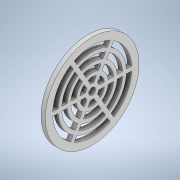
# Autodesk Inventor part: flat drain cover
Saved by Autodesk Inventor 2020.4 (Build 244396000, 396)
## iProperties
Created: 2023-07-18
Part Number: flat drain cover
Material: Generic
Document SubType Name: Modeling
Designer: Paul
Density: 1 g/cm^3
Appearance: Default
Author: Paul
Autodesk Inventor part; units mm, degrees
ref_plane "YZ Plane" through (0, 0, 0) normal (1, 0, 0) x (0, 1, 0)
ref_plane "XZ Plane" through (0, 0, 0) normal (0, 1, 0) x (-1, 0, 0)
ref_plane "XY Plane" through (0, 0, 0) normal (0, 0, 1) x (1, 0, 0)
sketch "Sketch1" plane through (0, 0, 0) normal (0, 1, 0) x (-1, 0, 0)
  line L0 (0, 5.08) -> (0, 10.668)
  line L1 (0, 0) -> (0, 10.668) construction
  line L2 (0, 10.668) -> (0, 18.542)
  line L3 (0, 18.542) -> (0, 24.13)
  line L4 (0, 24.13) -> (0, 32.004)
  line L5 (0, 32.004) -> (0, 37.592)
  line L6 (0, 37.592) -> (0, 45.466)
  line L7 (0, 45.466) -> (0, 51.054)
  line L8 (0, 51.054) -> (0, 58.928)
  line L9 (0, 58.928) -> (0, 66.802)
  line L10 (0, 0) -> (8.7387, 6.1189) construction
  line L11 (0, 0) -> (0, 18.542) construction
  line L12 (0, 0) -> (0, 24.13) construction
  line L13 (0, 0) -> (0, 32.004) construction
  line L14 (0, 0) -> (0, 37.592) construction
  line L15 (0, 0) -> (0, 45.466) construction
  line L16 (0, 0) -> (0, 51.054) construction
  line L17 (0, 0) -> (0, 58.928) construction
  line L18 (0, 0) -> (0, 66.802) construction
  line L19 (0, 0) -> (69.85, 0) construction
  line L20 (0, 0) -> (69.85, 0) construction
  line L21 (0, 66.802) -> (0, 69.85)
  line L22 (0, 0) -> (0, 5.08)
  line L23 (0, 69.85) -> (6.35, 69.85)
  line L24 (6.35, 69.85) -> (6.35, 0)
  line L25 (0, 5.08) -> (6.35, 5.08)
  line L26 (0, 10.668) -> (6.35, 10.668)
  line L27 (0, 18.542) -> (6.35, 18.542)
  line L28 (0, 24.13) -> (6.35, 24.13)
  line L29 (0, 32.004) -> (6.35, 32.004)
  line L30 (0, 37.592) -> (6.35, 37.592)
  line L31 (0, 45.466) -> (6.35, 45.466)
  line L32 (0, 51.054) -> (6.35, 51.054)
  line L33 (0, 58.928) -> (6.35, 58.928)
  dimension "d2" = 5.588
  dimension "d4" = 7.874
  dimension "d5" = 5.588
  dimension "d6" = 7.874
  dimension "d7" = 5.588
  dimension "d8" = 7.874
  dimension "d9" = 5.588
  dimension "d10" = 7.874
  dimension "d11" = 7.874
  dimension "d24" = 5.08
  dimension "d25" = 6.35
  dimension "d26" = 3.048
  constraints: 66 end point, 12 horizontal, 10 coincident, 6 point on line, 4 vertical, 1 collinear, 1 parallel, 12 other
  measures "d2" distance of L0.start L0.end
  measures "d4" distance of L0.end L2.end
  measures "d5" distance of L2.end L3.end
  measures "d6" distance of L3.end L4.end
  measures "d7" distance of L4.end L5.end
  measures "d8" distance of L5.end L6.end
  measures "d9" distance of L6.end L7.end
  measures "d10" distance of L7.end L8.end
  measures "d11" distance of L8.end L9.end
  measures "d24" distance of L22.start L0.start
  measures "d25" distance of L21.end L23.end
  measures "d26" distance of L9.end L21.end
revolve "Revolution1" add sketch "Sketch1" angle 360 about axis through (0, 0, 0) along (-1, 0, 0) contours L0 L26 L24 L25 | L3 L28 L24 L27 | L5 L30 L24 L29 | L7 L32 L24 L31 | L9 L21 L23 L24 L33
sketch "Sketch2" plane through (-6.35, 0, 0) normal (-1, 0, 0) x (0, 0, 1)
  line L0 (69.6277, 3.175) -> (-69.6277, 3.175)
  line L1 (-69.6277, 3.175) -> (-69.6277, -3.175)
  line L2 (-69.6277, -3.175) -> (69.6277, -3.175)
  line L3 (69.6277, -3.175) -> (69.6277, 3.175)
  circle A0 centre (0, 0) radius 5.08 projected
  line L4 (69.6277, 3.175) -> (-69.6277, -3.175) construction
  line L5 (-69.6277, 3.175) -> (69.6277, -3.175) construction
  line L6 (32.0642, 61.8868) -> (-37.5635, -58.7118)
  line L7 (-32.0642, -61.8868) -> (37.5635, 58.7118)
  line L8 (-37.5635, -58.7118) -> (-32.0642, -61.8868)
  line L9 (37.5635, 58.7118) -> (32.0642, 61.8868)
  line L10 (37.5635, -58.7118) -> (-32.0642, 61.8868)
  line L11 (-37.5635, 58.7118) -> (32.0642, -61.8868)
  line L12 (-32.0642, 61.8868) -> (-37.5635, 58.7118)
  line L13 (32.0642, -61.8868) -> (37.5635, -58.7118)
  point P0 (-5.4993, 3.175)
  point P1 (-5.4993, -3.175)
  point P2 (0, -6.35)
  point P3 (5.4993, -3.175)
  point P4 (5.4993, 3.175)
  point P5 (0, 6.35)
  dimension "d28" = 6.35
  dimension "d31" = 360
  constraints: 28 end point, 2 coincident, 2 midpoint, 2 parallel, 1 horizontal, 1 perpendicular, 26 other
  measures "d28" distance of L1.end L0.end
extrude "Extrusion1" add sketch "Sketch2" against normal blind 6.35
sketch "Sketch3" plane through (0, 0, 0) normal (1, 0, 0) x (0, 0, -1)
  circle A0 centre (0, 0) radius 5.08
  dimension "d35" = 10.16
  constraints: 1 centre point, 1 coincident
  measures "d35" diameter of A0
extrude "Extrusion2" cut sketch "Sketch3" against normal blind 25.4
equation "\"d2\" = PR"
equation "\"d4\" = HR"
equation "\"d5\" = PR"
equation "\"d6\" = HR"
equation "\"d7\" = PR"
equation "\"d8\" = HR"
equation "\"d9\" = PR"
equation "\"d10\" = HR"
equation "\"d11\" = HR"
equation "\"HR\" = 7.874"
equation "\"PR\" = 5.588"
equation "\"HA\" = 55deg"
body "Solid1"
